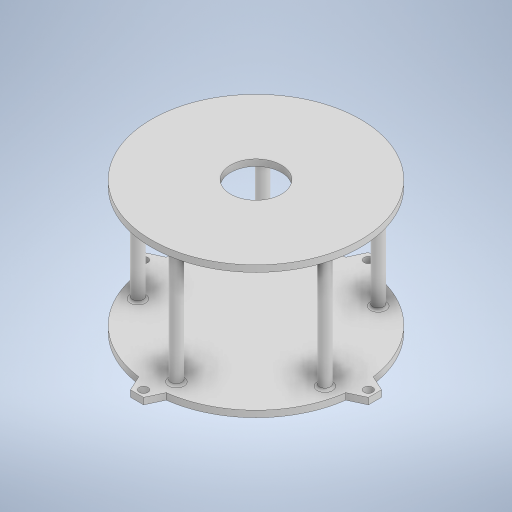
# Autodesk Inventor part: Pieza_base_1
Saved by Autodesk Inventor 2023 (Build 270158000, 158)
## iProperties
Created: 2024-09-21
Part Number: Pieza_base_1
Material: Genérico
Document SubType Name: Sheet Metal
Designer: sebas
Density: 1 g/cm^3
Sheet Metal Rule: Por defecto_mm
Appearance: Valor por defecto
Author: sebas
Autodesk Inventor part; units mm, degrees
ref_plane "YZ Plane" through (0, 0, 0) normal (1, 0, 0) x (0, 1, 0)
ref_plane "XZ Plane" through (0, 0, 0) normal (0, 1, 0) x (-1, 0, 0)
sketch "Boceto1" plane through (0, 0, 0) normal (0, 1, 0) x (-1, 0, 0)
  circle A0 centre (0, 0) radius 47.85
  dimension "d0" = 95.7
  constraints: 1 centre point, 1 coincident
  measures "d0" diameter of A0
extrude "Extrusión1" add sketch "Boceto1" along normal blind 2.96
ref_plane "Plano de trabajo1" through (0, 57.66, 0) normal (0, 1, 0) x (1, 0, 0)
sketch "Boceto2" plane through (0, 57.66, 0) normal (0, 1, 0) x (1, 0, 0)
  circle A0 centre (0, 0) radius 47.85 projected
extrude "Extrusión2" add sketch "Boceto2" along normal blind 2.96
sketch "Boceto3" plane through (0, 0, 0) normal (0, -1, 0) x (1, 0, 0)
  circle A0 centre (0, 0) radius 51.5 construction
  circle A1 centre (51.5, 0) radius 2
  line L0 (47.4341, 6.2949) -> (54.5, 3)
  line L1 (54.5, 3) -> (54.5, -3)
  line L2 (54.5, -3) -> (47.4341, -6.2949)
  line L3 (0, 0) -> (0, 96) construction
  line L4 (51.5, 0) -> (55.6486, 0) construction
  arc A2 (47.4341, -6.2949) -> (47.4341, 6.2949) centre (0, 0) ccw
  dimension "d6" = 103
  dimension "d7" = 4
  dimension "d8" = 115
  dimension "d9" = 115
  dimension "d10" = 3
  dimension "d11" = 6
  constraints: 10 end point, 4 point on circle, 3 centre point, 2 coincident, 2 vertical, 1 horizontal, 1 symmetric about line
  measures "d6" diameter of A0
  measures "d7" diameter of A1
  measures "d8" angle of L1 L0
  measures "d9" angle of L2 L1
  measures "d10" distance from line of L1 A1.centre
  measures "d11" distance of L0.end L1.end
extrude "Extrusión3" add sketch "Boceto3" against normal blind 2.96
pattern_circular "Patrón circular1" count 4 over 360 about axis through (0, -10, 0) along (0, 1, 0) of "Extrusión3"
sketch "Boceto4" plane through (0, 0, 0) normal (0, -1, 0) x (1, 0, 0)
  circle A0 centre (0, 0) radius 41 construction
  line L0 (0, 0) -> (20.5, -35.507) construction
  line L1 (0, 0) -> (0, -41) construction
  circle A1 centre (20.5, -35.507) radius 2.5
  dimension "d17" = 82
  dimension "d18" = 30
  dimension "d19" = 5
  constraints: 4 end point, 2 centre point, 2 coincident, 2 point on circle, 1 vertical
  measures "d17" diameter of A0
  measures "d18" angle of L1 L0
  measures "d19" diameter of A1
extrude "Extrusión4" add sketch "Boceto4" against normal up to surface (60.62 mm away)
fillet "Empalme1" radius 1 2 edges at (18, 57.66, -35.507) (18, 2.96, -35.507)
pattern_circular "Patrón circular2" count 5 over 360 about axis through (0, -10, 0) along (0, 1, 0) of "Extrusión4", "Empalme1"
sketch "Boceto5" plane through (0, 60.62, 0) normal (0, 1, 0) x (1, 0, 0)
  circle A0 centre (0, 0) radius 11.6
  dimension "d26" = 23.2
  constraints: 1 centre point, 1 coincident
  measures "d26" diameter of A0
extrude "Extrusión5" cut sketch "Boceto5" against normal up to surface (2.96 mm away)
sketch "Boceto6" plane through (0, 0, 0) normal (0, -1, 0) x (1, 0, 0)
  line L0 (25.2929, 5) -> (25.2929, -33.3087) construction
  line L1 (25.2929, -33.3087) -> (6, -33.3087) construction
  line L2 (6, -33.3087) -> (6, 5) construction
  line L3 (6, 5) -> (25.2929, 5) construction
  line L4 (13.254, -2.6726) -> (13.254, 3.1815)
  line L5 (13.254, 3.1815) -> (14.4793, 3.1815)
  line L6 (14.4793, 3.1815) -> (14.4793, 1.0032)
  line L7 (14.4793, 1.0032) -> (22.5214, 1.0032)
  line L8 (22.5214, 1.0032) -> (22.5214, 3.1815)
  line L9 (22.5214, 3.1815) -> (23.6203, 3.1815)
  spline S0 degree 2 poles (23.6203, 3.1815) (23.6203, 1.9465) (24.3204, 0.7796) (25.2929, 0.7018) knots 0 0 0 1 2 2 2
  line L10 (25.2929, 0.7018) -> (25.2929, -0.5429)
  line L11 (25.2929, -0.5429) -> (14.4793, -0.5429)
  line L12 (14.4793, -0.5429) -> (14.4793, -2.6726)
  line L13 (14.4793, -2.6726) -> (13.254, -2.6726)
  point P0 (0, 0)
  constraints: 2 other
extrude "Extrusión6" cut sketch "Boceto6" against normal blind 0.5
equation "\"Radio_pliegue\" = Grosor"
equation "\"Anchura_desahogo_plegado\" = Grosor"
equation "\"Profundidad_desahogo_plegado\" = 0.5 * Grosor"
equation "\"Tamaño_destalonado\" = 4 * Grosor"
equation "\"Remanente_mínimo\" = 2 * Grosor"
equation "\"Radiodetransición\" = Radio_pliegue"
equation "\"Tamaño_de_radio_de_Jacobi\" = Radio_pliegue"
equation "\"TamañoSeparación\" = Grosor"
equation "\"Grosor\" = 0.5"
